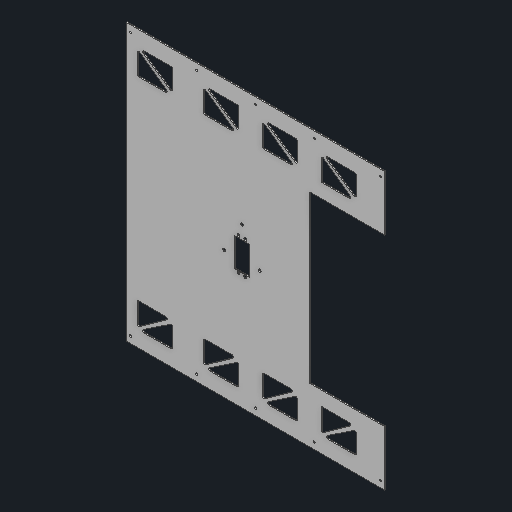
# Autodesk Inventor part: ВЕРХ 25-26
Saved by Autodesk Inventor 2026.2 (Build 302298000, 298)
## iProperties
Created: 2025-09-28
Part Number: ВЕРХ 25-26
Material: Типовые
Document SubType Name: Modeling
Designer: GameHD
Density: 1 g/cm^3
Appearance: По умолчанию
Author: GameHD
Autodesk Inventor part; units mm, degrees
(part 1 of 2)
ref_plane "YZ Plane" through (0, 0, 0) normal (1, 0, 0) x (0, 1, 0)
ref_plane "XZ Plane" through (0, 0, 0) normal (0, 1, 0) x (-1, 0, 0)
ref_plane "XY Plane" through (0, 0, 0) normal (0, 0, 1) x (1, 0, 0)
sketch "Эскиз1" plane through (0, 0, 0) normal (0, 0, 1) x (1, 0, 0)
  line L0 (0, 0) -> (380, 0)
  line L1 (380, 0) -> (380, 406)
  line L2 (380, 406) -> (0, 406)
  line L3 (0, 406) -> (0, 0)
  circle A0 centre (189.9999, 9.5) radius 1.625
  circle A1 centre (276.4236, 9.5) radius 1.625
  circle A2 centre (103.5763, 9.5) radius 1.625
  circle A3 centre (373.8998, 9.5) radius 1.625
  circle A4 centre (6.1, 9.5) radius 1.625
  line L4 (0, -31.725) -> (0, 41.275)
  line L5 (0, 203) -> (417.5125, 203)
  circle A5 centre (189.9999, 396.5) radius 1.625
  circle A6 centre (276.4236, 396.5) radius 1.625
  circle A7 centre (373.8998, 396.5) radius 1.625
  circle A8 centre (103.5763, 396.5) radius 1.625
  circle A9 centre (6.1, 396.5) radius 1.625
  circle A10 centre (189.9999, -129.0468) radius 1.625
  circle A11 centre (276.4236, -129.0468) radius 1.625
  circle A12 centre (373.8998, -129.0468) radius 1.625
  circle A13 centre (103.5763, -129.0468) radius 1.625
  circle A14 centre (6.1, -129.0468) radius 1.625
  circle A15 centre (189.9999, 535.0468) radius 1.625
  circle A16 centre (103.5763, 535.0468) radius 1.625
  circle A17 centre (373.8998, 535.0468) radius 1.625
  circle A18 centre (6.1, 535.0468) radius 1.625
  circle A19 centre (276.4236, 535.0468) radius 1.625
  line L6 (380, 203) -> (280, 203)
  line L7 (280, 203) -> (280, 81)
  line L8 (280, 81) -> (380, 81)
  line L9 (380, 81) -> (380, 203)
  line L10 (280, 203) -> (280, 325)
  line L11 (280, 325) -> (380, 325)
  circle A20 centre (6.1, 198.6) radius 1.625 projected
  arc A21 (257.5001, 181.25) -> (253.5001, 185.25) centre (253.5001, 181.25) ccw projected
  line L12 (253.5001, 185.25) -> (186.5001, 185.25) projected
  arc A22 (186.5001, 185.25) -> (182.5001, 181.25) centre (186.5001, 181.25) ccw projected
  line L13 (182.5001, 181.25) -> (182.5001, 139.25) projected
  arc A23 (182.5001, 139.25) -> (186.5001, 135.25) centre (186.5001, 139.25) ccw projected
  line L14 (186.5001, 135.25) -> (253.5001, 135.25) projected
  arc A24 (253.5001, 135.25) -> (257.5001, 139.25) centre (253.5001, 139.25) ccw projected
  line L15 (257.5001, 139.25) -> (257.5001, 181.25) projected
  line L16 (253.5001, -135.25) -> (186.5001, -135.25) projected
  arc A25 (186.5001, -135.25) -> (182.5001, -139.25) centre (186.5001, -139.25) ccw projected
  line L17 (182.5001, -139.25) -> (182.5001, -181.25) projected
  arc A26 (182.5001, -181.25) -> (186.5001, -185.25) centre (186.5001, -181.25) ccw projected
  line L18 (186.5001, -185.25) -> (253.5001, -185.25) projected
  arc A27 (253.5001, -185.25) -> (257.5001, -181.25) centre (253.5001, -181.25) ccw projected
  line L19 (257.5001, -181.25) -> (257.5001, -139.25) projected
  arc A28 (257.5001, -139.25) -> (253.5001, -135.25) centre (253.5001, -139.25) ccw projected
  arc A29 (148.6202, 128.9218) -> (145.3798, 128.9218) centre (147, 129.0468) ccw projected
  arc A30 (145.3798, 128.9218) -> (148.6202, 128.9218) centre (147, 128.7968) ccw projected
  arc A31 (371.3798, 111.6718) -> (374.6202, 111.6718) centre (373, 111.5468) ccw projected
  arc A32 (374.6202, 111.6718) -> (371.3798, 111.6718) centre (373, 111.7968) ccw projected
  arc A33 (231.3798, -128.9218) -> (234.6202, -128.9218) centre (233, -129.0468) ccw projected
  arc A34 (234.6202, -128.9218) -> (231.3798, -128.9218) centre (233, -128.7968) ccw projected
  arc A35 (5.38, -128.9218) -> (8.6204, -128.9218) centre (7.0002, -129.0468) ccw projected
  arc A36 (8.6204, -128.9218) -> (5.38, -128.9218) centre (7.0002, -128.7968) ccw projected
  arc A37 (148.6202, -111.6718) -> (145.3798, -111.6718) centre (147, -111.5468) ccw projected
  arc A38 (145.3798, -111.6718) -> (148.6202, -111.6718) centre (147, -111.7968) ccw projected
  arc A39 (374.6202, -111.6718) -> (371.3798, -111.6718) centre (373, -111.5468) ccw projected
  arc A40 (371.3798, -111.6718) -> (374.6202, -111.6718) centre (373, -111.7968) ccw projected
  arc A41 (231.3798, 111.6718) -> (234.6202, 111.6718) centre (233, 111.5468) ccw projected
  arc A42 (234.6202, 111.6718) -> (231.3798, 111.6718) centre (233, 111.7968) ccw projected
  arc A43 (5.38, 111.6718) -> (8.6204, 111.6718) centre (7.0002, 111.5468) ccw projected
  arc A44 (8.6204, 111.6718) -> (5.38, 111.6718) centre (7.0002, 111.7968) ccw projected
  arc A45 (145.3798, 111.6718) -> (148.6202, 111.6718) centre (147, 111.5468) ccw projected
  arc A46 (148.6202, 111.6718) -> (145.3798, 111.6718) centre (147, 111.7968) ccw projected
  arc A47 (374.6202, 128.9218) -> (371.3798, 128.9218) centre (373, 129.0468) ccw projected
  arc A48 (371.3798, 128.9218) -> (374.6202, 128.9218) centre (373, 128.7968) ccw projected
  arc A49 (234.6202, -111.6718) -> (231.3798, -111.6718) centre (233, -111.5468) ccw projected
  arc A50 (231.3798, -111.6718) -> (234.6202, -111.6718) centre (233, -111.7968) ccw projected
  arc A51 (8.6204, -111.6718) -> (5.38, -111.6718) centre (7.0002, -111.5468) ccw projected
  arc A52 (5.38, -111.6718) -> (8.6204, -111.6718) centre (7.0002, -111.7968) ccw projected
  arc A53 (145.3798, -128.9218) -> (148.6202, -128.9218) centre (147, -129.0468) ccw projected
  arc A54 (148.6202, -128.9218) -> (145.3798, -128.9218) centre (147, -128.7968) ccw projected
  arc A55 (371.3798, -128.9218) -> (374.6202, -128.9218) centre (373, -129.0468) ccw projected
  arc A56 (374.6202, -128.9218) -> (371.3798, -128.9218) centre (373, -128.7968) ccw projected
  arc A57 (234.6202, 128.9218) -> (231.3798, 128.9218) centre (233, 129.0468) ccw projected
  arc A58 (231.3798, 128.9218) -> (234.6202, 128.9218) centre (233, 128.7968) ccw projected
  arc A59 (8.6204, 128.9218) -> (5.38, 128.9218) centre (7.0002, 129.0468) ccw projected
  arc A60 (5.38, 128.9218) -> (8.6204, 128.9218) centre (7.0002, 128.7968) ccw projected
  circle A61 centre (373.9, 198.6) radius 1.625 projected
  circle A62 centre (374, -198.6) radius 1.625 projected
  circle A63 centre (6.1, 198.6) radius 1.625 projected
  circle A64 centre (6.1, -198.6) radius 1.625 projected
  circle A65 centre (190.0848, 193.5) radius 1.625 projected
  circle A66 centre (190.0848, -193.5) radius 1.625 projected
  circle A67 centre (233, 193.5) radius 1.625 projected
  circle A68 centre (233, -193.5) radius 1.625 projected
  circle A69 centre (134.0059, -1.825) radius 1.85 projected
  arc A70 (197.7028, 0) -> (198.309, 0) centre (198.0059, -1.825) ccw projected
  line L20 (198.309, 0) -> (197.7028, 0) projected
  circle A71 centre (134.0059, -60.625) radius 2 projected
  circle A72 centre (317.9941, 32.25) radius 2.1 projected
  circle A73 centre (62.0059, -32.25) radius 2.1 projected
  circle A74 centre (123.0059, -32.25) radius 2.1 projected
  circle A75 centre (317.9941, -32.25) radius 2.1 projected
  circle A76 centre (256.9941, 32.25) radius 2.1 projected
  circle A77 centre (62.0059, 32.25) radius 2.1 projected
  circle A78 centre (123.0059, 32.25) radius 2.1 projected
  circle A79 centre (256.9941, -32.25) radius 2.1 projected
  line L21 (49, -20) -> (13, -20) projected
  arc A80 (13, -20) -> (10, -23) centre (13, -23) ccw projected
  line L22 (10, -23) -> (10, -89) projected
  arc A81 (10, -89) -> (13, -92) centre (13, -89) ccw projected
  line L23 (13, -92) -> (49, -92) projected
  arc A82 (49, -92) -> (52, -89) centre (49, -89) ccw projected
  line L24 (52, -89) -> (52, -23) projected
  arc A83 (52, -23) -> (49, -20) centre (49, -23) ccw projected
  circle A84 centre (170.0002, 134.1128) radius 2.1 projected
  circle A85 centre (61.343, 102) radius 2.1 projected
  circle A86 centre (170.0002, -134.1128) radius 2.1 projected
  circle A87 centre (61.343, -11.0092) radius 2.1 projected
  circle A88 centre (65, -49.75) radius 2.1 projected
  circle A89 centre (65, -82) radius 2.1 projected
  arc A90 (32.152, -145) -> (34.152, -143) centre (32.152, -143) ccw projected
  line L25 (32.152, -145) -> (8, -145) projected
  arc A91 (8, -145) -> (5, -148) centre (8, -148) ccw projected
  line L26 (5, -148) -> (5, -192) projected
  arc A92 (5, -192) -> (8, -195) centre (8, -192) ccw projected
  line L27 (8, -195) -> (165, -195) projected
  arc A93 (165, -195) -> (168, -192) centre (165, -192) ccw projected
  line L28 (168, -192) -> (168, -148) projected
  arc A94 (168, -148) -> (165, -145) centre (165, -148) ccw projected
  line L29 (165, -145) -> (116.152, -145) projected
  arc A95 (114.152, -143) -> (116.152, -145) centre (116.152, -143) ccw projected
  line L30 (114.152, -143) -> (114.152, -131) projected
  arc A96 (114.152, -131) -> (112.152, -129) centre (112.152, -131) ccw projected
  line L31 (112.152, -129) -> (36.152, -129) projected
  arc A97 (36.152, -129) -> (34.152, -131) centre (36.152, -131) ccw projected
  line L32 (34.152, -131) -> (34.152, -143) projected
  arc A98 (345.848, -143) -> (347.848, -145) centre (347.848, -143) ccw projected
  line L33 (345.848, -143) -> (345.848, -131) projected
  arc A99 (345.848, -131) -> (343.848, -129) centre (343.848, -131) ccw projected
  line L34 (343.848, -129) -> (267.848, -129) projected
  arc A100 (267.848, -129) -> (265.848, -131) centre (267.848, -131) ccw projected
  line L35 (265.848, -131) -> (265.848, -193) projected
  arc A101 (265.848, -193) -> (267.848, -195) centre (267.848, -193) ccw projected
  line L36 (267.848, -195) -> (372, -195) projected
  arc A102 (372, -195) -> (375, -192) centre (372, -192) ccw projected
  line L37 (375, -192) -> (375, -148) projected
  arc A103 (375, -148) -> (372, -145) centre (372, -148) ccw projected
  line L38 (372, -145) -> (347.848, -145) projected
  arc A104 (347.848, 145) -> (345.848, 143) centre (347.848, 143) ccw projected
  line L39 (347.848, 145) -> (372, 145) projected
  arc A105 (372, 145) -> (375, 148) centre (372, 148) ccw projected
  line L40 (375, 148) -> (375, 192) projected
  arc A106 (375, 192) -> (372, 195) centre (372, 192) ccw projected
  line L41 (372, 195) -> (267.848, 195) projected
  arc A107 (267.848, 195) -> (265.848, 193) centre (267.848, 193) ccw projected
  line L42 (265.848, 193) -> (265.848, 131) projected
  arc A108 (265.848, 131) -> (267.848, 129) centre (267.848, 131) ccw projected
  line L43 (267.848, 129) -> (343.848, 129) projected
  arc A109 (343.848, 129) -> (345.848, 131) centre (343.848, 131) ccw projected
  line L44 (345.848, 131) -> (345.848, 143) projected
  arc A110 (34.152, 143) -> (32.152, 145) centre (32.152, 143) ccw projected
  line L45 (34.152, 143) -> (34.152, 131) projected
  arc A111 (34.152, 131) -> (36.152, 129) centre (36.152, 131) ccw projected
  line L46 (36.152, 129) -> (112.152, 129) projected
  arc A112 (112.152, 129) -> (114.152, 131) centre (112.152, 131) ccw projected
  line L47 (114.152, 131) -> (114.152, 143) projected
  arc A113 (116.152, 145) -> (114.152, 143) centre (116.152, 143) ccw projected
  line L48 (116.152, 145) -> (165, 145) projected
  arc A114 (165, 145) -> (168, 148) centre (165, 148) ccw projected
  line L49 (168, 148) -> (168, 192) projected
  arc A115 (168, 192) -> (165, 195) centre (165, 192) ccw projected
  line L50 (165, 195) -> (8, 195) projected
  arc A116 (8, 195) -> (5, 192) centre (8, 192) ccw projected
  line L51 (5, 192) -> (5, 148) projected
  arc A117 (5, 148) -> (8, 145) centre (8, 148) ccw projected
  line L52 (8, 145) -> (32.152, 145) projected
  line L53 (176.1539, 5.9063) -> (141.4028, 21.6949) projected
  arc A118 (141.4028, 21.6949) -> (137.8279, 17.0788) centre (140.1619, 18.9636) ccw projected
  line L54 (137.8279, 17.0788) -> (150.5778, 1.2902) projected
  arc A119 (150.5778, 1.2902) -> (152.9118, 0.175) centre (152.9118, 3.175) ccw projected
  line L55 (152.9118, 0.175) -> (174.913, 0.175) projected
  arc A120 (174.913, 0.175) -> (176.1539, 5.9063) centre (174.913, 3.175) ccw projected
  line L56 (164.9717, -29.4592) -> (165.9394, -28.5702) projected
  arc A121 (165.9394, -28.5702) -> (166.2437, -24.4762) centre (163.9097, -26.361) ccw projected
  line L57 (166.2437, -24.4762) -> (150.4677, -4.9402) projected
  arc A122 (150.4677, -4.9402) -> (148.1337, -3.825) centre (148.1337, -6.825) ccw projected
  line L58 (148.1337, -3.825) -> (145.4623, -3.825) projected
  arc A123 (145.4623, -3.825) -> (142.7128, -5.625) centre (145.4623, -6.825) ccw projected
  arc A124 (137.8059, -10.5319) -> (142.7128, -5.625) centre (134.0059, -1.825) ccw projected
  arc A125 (137.8059, -10.5319) -> (136.0059, -13.2814) centre (139.0059, -13.2814) ccw projected
  line L59 (136.0059, -13.2814) -> (136.0059, -27.25) projected
  arc A126 (136.0059, -27.25) -> (139.0059, -30.25) centre (139.0059, -27.25) ccw projected
  line L60 (139.0059, -30.25) -> (162.942, -30.25) projected
  arc A127 (162.942, -30.25) -> (164.9717, -29.4592) centre (162.942, -27.25) ccw projected
  line L61 (190.9762, -10.9995) -> (175.6931, -25.0408) projected
  arc A128 (175.6931, -25.0408) -> (177.7227, -30.25) centre (177.7227, -27.25) ccw projected
  line L62 (177.7227, -30.25) -> (193.0059, -30.25) projected
  arc A129 (193.0059, -30.25) -> (196.0059, -27.25) centre (193.0059, -27.25) ccw projected
  line L63 (196.0059, -27.25) -> (196.0059, -13.2086) projected
  arc A130 (196.0059, -13.2086) -> (190.9762, -10.9995) centre (193.0059, -13.2086) ccw projected
  line L64 (75.0034, -76.8076) -> (112.8628, -65.0804) projected
  arc A131 (112.8628, -65.0804) -> (112.4422, -59.2513) centre (111.9752, -62.2148) ccw projected
  line L65 (112.4422, -59.2513) -> (74.5828, -53.2849) projected
  arc A132 (74.5828, -53.2849) -> (71.1158, -56.2483) centre (74.1158, -56.2483) ccw projected
  line L66 (71.1158, -56.2483) -> (71.1158, -73.942) projected
  arc A133 (71.1158, -73.942) -> (75.0034, -76.8076) centre (74.1158, -73.942) ccw projected
  line L67 (273.1271, 34.25) -> (305.3345, 34.25) projected
  arc A134 (305.3345, 34.25) -> (307.3845, 39.4403) centre (305.3345, 37.25) ccw projected
  line L68 (307.3845, 39.4403) -> (293.7654, 52.1866) projected
  arc A135 (293.7654, 52.1866) -> (290.0188, 52.4704) centre (291.7154, 49.9963) ccw projected
  line L69 (290.0188, 52.4704) -> (271.4305, 39.7242) projected
  arc A136 (271.4305, 39.7242) -> (273.1271, 34.25) centre (273.1271, 37.25) ccw projected
  line L70 (237.7677, -24.5838) -> (207.2709, -8.8541) projected
  arc A137 (207.2709, -8.8541) -> (204.0022, -9.1935) centre (205.8957, -11.5203) ccw projected
  arc A138 (201.8059, -10.5319) -> (204.0022, -9.1935) centre (198.0059, -1.825) ccw projected
  arc A139 (201.8059, -10.5319) -> (200.0059, -13.2814) centre (203.0059, -13.2814) ccw projected
  line L71 (200.0059, -13.2814) -> (200.0059, -27.25) projected
  arc A140 (200.0059, -27.25) -> (203.0059, -30.25) centre (203.0059, -27.25) ccw projected
  line L72 (203.0059, -30.25) -> (236.3925, -30.25) projected
  arc A141 (236.3925, -30.25) -> (237.7677, -24.5838) centre (236.3925, -27.25) ccw projected
  line L73 (171.7502, 96.3659) -> (188.242, 84.4391) projected
  arc A142 (188.242, 84.4391) -> (191.758, 84.4391) centre (190, 86.8701) ccw projected
  line L74 (191.758, 84.4391) -> (215.7595, 101.7968) projected
  line L75 (215.7595, 101.7968) -> (173.5082, 101.7968) projected
  arc A143 (173.5082, 101.7968) -> (171.7502, 96.3659) centre (173.5082, 98.7968) ccw projected
  line L76 (265.3115, 40.3784) -> (285.9348, 54.5201) projected
  arc A144 (285.9348, 54.5201) -> (286.2882, 59.1846) centre (284.2382, 56.9942) ccw projected
  line L77 (286.2882, 59.1846) -> (245.2049, 97.6348) projected
  arc A145 (245.2049, 97.6348) -> (240.2828, 94.5781) centre (243.1549, 95.4444) ccw projected
  line L78 (240.2828, 94.5781) -> (255.6005, 43.7959) projected
  arc A146 (255.6005, 43.7959) -> (258.1178, 41.6833) centre (258.4726, 44.6622) ccw projected
  arc A147 (262.0259, 40.308) -> (258.1178, 41.6833) centre (256.9941, 32.25) ccw projected
  arc A148 (262.0259, 40.308) -> (265.3115, 40.3784) centre (263.6149, 42.8526) ccw projected
  arc A149 (72.6155, 39.4403) -> (74.6655, 34.25) centre (74.6655, 37.25) ccw projected
  line L79 (74.6655, 34.25) -> (111.9119, 34.25) projected
  arc A150 (111.9119, 34.25) -> (114.1595, 39.237) centre (111.9119, 37.25) ccw projected
  line L80 (114.1595, 39.237) -> (97.2953, 58.3129) projected
  arc A151 (97.2953, 58.3129) -> (92.9977, 58.5163) centre (95.0477, 56.3259) ccw projected
  line L81 (92.9977, 58.5163) -> (72.6155, 39.4403) projected
  line L82 (252.1574, 96.6064) -> (290.6344, 60.5955) projected
  arc A152 (290.6344, 60.5955) -> (294.3809, 60.3117) centre (292.6843, 62.7859) ccw projected
  line L83 (294.3809, 60.3117) -> (316.6907, 75.6098) projected
  arc A153 (316.6907, 75.6098) -> (317.9941, 78.084) centre (314.9941, 78.084) ccw projected
  line L84 (317.9941, 78.084) -> (317.9941, 98.7968) projected
  arc A154 (317.9941, 98.7968) -> (314.9941, 101.7968) centre (314.9941, 98.7968) ccw projected
  line L85 (314.9941, 101.7968) -> (254.2074, 101.7968) projected
  arc A155 (254.2074, 101.7968) -> (252.1574, 96.6064) centre (254.2074, 98.7968) ccw projected
  line L86 (196.7743, 78.2686) -> (212.8517, 66.6416) projected
  arc A156 (212.8517, 66.6416) -> (217.4768, 68.1895) centre (214.6097, 69.0726) ccw projected
  line L87 (217.4768, 68.1895) -> (226.6315, 97.9138) projected
  arc A157 (226.6315, 97.9138) -> (223.7644, 101.7968) centre (223.7644, 98.7968) ccw projected
  line L88 (223.7644, 101.7968) -> (223.5564, 101.7968) projected
  arc A158 (223.5564, 101.7968) -> (221.7984, 101.2277) centre (223.5564, 98.7968) ccw projected
  line L89 (221.7984, 101.2277) -> (196.7743, 83.1305) projected
  arc A159 (196.7743, 83.1305) -> (196.7743, 78.2686) centre (198.5323, 80.6996) ccw projected
  line L90 (209.1045, -5.2991) -> (247.729, -25.2209) projected
  arc A160 (247.729, -25.2209) -> (250.9978, -24.8815) centre (249.1042, -22.5547) ccw projected
  arc A161 (253.1941, -23.5431) -> (250.9978, -24.8815) centre (256.9941, -32.25) ccw projected
  arc A162 (253.1941, -23.5431) -> (254.9941, -20.7936) centre (251.9941, -20.7936) ccw projected
  line L91 (254.9941, -20.7936) -> (254.9941, 20.7936) projected
  arc A163 (254.9941, 20.7936) -> (253.1941, 23.5431) centre (251.9941, 20.7936) ccw projected
  arc A164 (251.3555, 24.6044) -> (253.1941, 23.5431) centre (256.9941, 32.25) ccw projected
  arc A165 (251.3555, 24.6044) -> (248.0743, 24.7877) centre (249.5749, 22.1899) ccw projected
  line L92 (248.0743, 24.7877) -> (208.9265, 2.1737) projected
  arc A166 (208.9265, 2.1737) -> (207.446, -0.7603) centre (210.4271, -0.424) ccw projected
  arc A167 (207.486, -2.439) -> (207.446, -0.7603) centre (198.0059, -1.825) ccw projected
  arc A168 (207.486, -2.439) -> (209.1045, -5.2991) centre (210.4797, -2.6329) ccw projected
  line L93 (290.6344, -60.5955) -> (250.0205, -98.6064) projected
  arc A169 (250.0205, -98.6064) -> (252.0705, -103.7968) centre (252.0705, -100.7968) ccw projected
  line L94 (252.0705, -103.7968) -> (314.9941, -103.7968) projected
  arc A170 (314.9941, -103.7968) -> (317.9941, -100.7968) centre (314.9941, -100.7968) ccw projected
  line L95 (317.9941, -100.7968) -> (317.9941, -78.084) projected
  arc A171 (317.9941, -78.084) -> (316.6907, -75.6098) centre (314.9941, -78.084) ccw projected
  line L96 (316.6907, -75.6098) -> (294.3809, -60.3117) projected
  arc A172 (294.3809, -60.3117) -> (290.6344, -60.5955) centre (292.6843, -62.7859) ccw projected
  line L97 (258.9941, 19.6864) -> (258.9941, -19.6864) projected
  arc A173 (258.9941, -19.6864) -> (264.1737, -21.7477) centre (261.9941, -19.6864) ccw projected
  line L98 (264.1737, -21.7477) -> (282.7918, -2.0614) projected
  arc A174 (282.7918, -2.0614) -> (282.7918, 2.0614) centre (280.6122, 0) ccw projected
  line L99 (282.7918, 2.0614) -> (264.1737, 21.7477) projected
  arc A175 (264.1737, 21.7477) -> (258.9941, 19.6864) centre (261.9941, 19.6864) ccw projected
  line L100 (73.6488, -49.0883) -> (89.4125, -51.5726) projected
  arc A176 (89.4125, -51.5726) -> (90.9794, -45.8181) centre (89.8795, -48.6092) ccw projected
  line L101 (90.9794, -45.8181) -> (75.2157, -39.6057) projected
  arc A177 (75.2157, -39.6057) -> (71.1158, -42.3967) centre (74.1158, -42.3967) ccw projected
  line L102 (71.1158, -42.3967) -> (71.1158, -46.1249) projected
  arc A178 (71.1158, -46.1249) -> (73.6488, -49.0883) centre (74.1158, -46.1249) ccw projected
  line L103 (136.0059, -37.25) -> (136.0059, -49.2414) projected
  arc A179 (136.0059, -49.2414) -> (141.0355, -51.4505) centre (139.0059, -49.2414) ccw projected
  line L104 (141.0355, -51.4505) -> (154.0874, -39.4592) projected
  arc A180 (154.0874, -39.4592) -> (152.0577, -34.25) centre (152.0577, -37.25) ccw projected
  line L105 (152.0577, -34.25) -> (139.0059, -34.25) projected
  arc A181 (139.0059, -34.25) -> (136.0059, -37.25) centre (139.0059, -37.25) ccw projected
  line L106 (187.6976, 26.0214) -> (194.3962, 11.0995) projected
  arc A182 (194.3962, 11.0995) -> (200.0002, 11.4451) centre (197.1331, 12.3281) ccw projected
  line L107 (200.0002, 11.4451) -> (204.5959, 26.367) projected
  arc A183 (204.5959, 26.367) -> (201.7288, 30.25) centre (201.7288, 27.25) ccw projected
  line L108 (201.7288, 30.25) -> (190.4345, 30.25) projected
  arc A184 (190.4345, 30.25) -> (187.6976, 26.0214) centre (190.4345, 27.25) ccw projected
  line L109 (96.148, -15.0552) -> (84.8346, -0.4618) projected
  arc A185 (84.8346, -0.4618) -> (80.7407, 0.156) centre (82.4637, -2.2999) ccw projected
  line L110 (80.7407, 0.156) -> (72.3928, -5.7004) projected
  arc A186 (72.3928, -5.7004) -> (71.1158, -8.1563) centre (74.1158, -8.1563) ccw projected
  line L111 (71.1158, -8.1563) -> (71.1158, -10.1207) projected
  arc A187 (71.1158, -10.1207) -> (73.1387, -12.9571) centre (74.1158, -10.1207) ccw projected
  line L112 (73.1387, -12.9571) -> (92.8, -19.7297) projected
  arc A188 (92.8, -19.7297) -> (96.148, -15.0552) centre (93.777, -16.8933) ccw projected
  line L113 (158.6531, -8.7098) -> (168.9546, -21.4664) projected
  arc A189 (168.9546, -21.4664) -> (173.3182, -21.7908) centre (171.2886, -19.5816) ccw projected
  line L114 (173.3182, -21.7908) -> (187.203, -9.0342) projected
  arc A190 (187.203, -9.0342) -> (185.1733, -3.825) centre (185.1733, -6.825) ccw projected
  line L115 (185.1733, -3.825) -> (160.9871, -3.825) projected
  arc A191 (160.9871, -3.825) -> (158.6531, -8.7098) centre (160.9871, -6.825) ccw projected
  line L116 (88.7233, 10.6423) -> (108.8956, 24.7941) projected
  arc A192 (108.8956, 24.7941) -> (107.1727, 30.25) centre (107.1727, 27.25) ccw projected
  line L117 (107.1727, 30.25) -> (74.1158, 30.25) projected
  arc A193 (74.1158, 30.25) -> (71.1158, 27.25) centre (74.1158, 27.25) ccw projected
  line L118 (71.1158, 27.25) -> (71.1158, 26.722) projected
  arc A194 (71.1158, 26.722) -> (71.9361, 24.6607) centre (74.1158, 26.722) ccw projected
  line L119 (71.9361, 24.6607) -> (84.8207, 11.0368) projected
  arc A195 (84.8207, 11.0368) -> (88.7233, 10.6423) centre (87.0003, 13.0982) ccw projected
  line L120 (138.452, 34.25) -> (174.984, 34.25) projected
  arc A196 (174.984, 34.25) -> (177.7209, 38.4786) centre (174.984, 37.25) ccw projected
  line L121 (177.7209, 38.4786) -> (168.7676, 58.4233) projected
  arc A197 (168.7676, 58.4233) -> (164.2727, 59.6256) centre (166.0307, 57.1947) ccw projected
  line L122 (164.2727, 59.6256) -> (136.694, 39.6809) projected
  arc A198 (136.694, 39.6809) -> (138.452, 34.25) centre (138.452, 37.25) ccw projected
  line L123 (183.2224, -39.1348) -> (190.6719, -48.3597) projected
  arc A199 (190.6719, -48.3597) -> (196.0059, -46.4749) centre (193.0059, -46.4749) ccw projected
  line L124 (196.0059, -46.4749) -> (196.0059, -37.25) projected
  arc A200 (196.0059, -37.25) -> (193.0059, -34.25) centre (193.0059, -37.25) ccw projected
  line L125 (193.0059, -34.25) -> (185.5564, -34.25) projected
  arc A201 (185.5564, -34.25) -> (183.2224, -39.1348) centre (185.5564, -37.25) ccw projected
  line L126 (104.4945, -94.2234) -> (129.3603, -103.259) projected
  arc A202 (129.3603, -103.259) -> (133.3849, -100.4394) centre (130.3849, -100.4394) ccw projected
  line L127 (133.3849, -100.4394) -> (133.3849, -94.0885) projected
  arc A203 (133.3849, -94.0885) -> (130.7069, -91.1058) centre (130.3849, -94.0885) ccw projected
  line L128 (130.7069, -91.1058) -> (105.8411, -88.4211) projected
  arc A204 (105.8411, -88.4211) -> (104.4945, -94.2234) centre (105.5191, -91.4038) ccw projected
  line L129 (266.425, 25.1886) -> (285.3145, 5.2154) projected
  arc A205 (285.3145, 5.2154) -> (289.6737, 5.2154) centre (287.4941, 7.2768) ccw projected
  line L130 (289.6737, 5.2154) -> (308.5632, 25.1886) projected
  arc A206 (308.5632, 25.1886) -> (306.3835, 30.25) centre (306.3835, 27.25) ccw projected
  line L131 (306.3835, 30.25) -> (268.6047, 30.25) projected
  arc A207 (268.6047, 30.25) -> (266.425, 25.1886) centre (268.6047, 27.25) ccw projected
  line L132 (76.1657, 48.2416) -> (90.4716, 61.6306) projected
  arc A208 (90.4716, 61.6306) -> (90.6693, 65.808) centre (88.4217, 63.821) ccw projected
  line L133 (90.6693, 65.808) -> (76.3634, 81.9901) projected
  arc A209 (76.3634, 81.9901) -> (71.1158, 80.0031) centre (74.1158, 80.0031) ccw projected
  line L134 (71.1158, 80.0031) -> (71.1158, 50.432) projected
  arc A210 (71.1158, 50.432) -> (76.1657, 48.2416) centre (74.1158, 50.432) ccw projected
  line L135 (133.824, 42.5418) -> (163.6065, 64.0802) projected
  arc A211 (163.6065, 64.0802) -> (164.5853, 67.7397) centre (161.8485, 66.5111) ccw projected
  line L136 (164.5853, 67.7397) -> (150.6579, 98.7648) projected
  arc A212 (150.6579, 98.7648) -> (145.0488, 98.4025) centre (147.921, 97.5362) ccw projected
  line L137 (145.0488, 98.4025) -> (129.1938, 45.8391) projected
  arc A213 (129.1938, 45.8391) -> (133.824, 42.5418) centre (132.066, 44.9727) ccw projected
  line L138 (71.8682, 93.1141) -> (93.4781, 68.6699) projected
  arc A214 (93.4781, 68.6699) -> (97.7757, 68.4666) centre (95.7258, 70.657) ccw projected
  line L139 (97.7757, 68.4666) -> (127.8426, 96.6064) projected
  arc A215 (127.8426, 96.6064) -> (125.7926, 101.7968) centre (125.7926, 98.7968) ccw projected
  line L140 (125.7926, 101.7968) -> (74.1158, 101.7968) projected
  arc A216 (74.1158, 101.7968) -> (71.1158, 98.7968) centre (74.1158, 98.7968) ccw projected
  line L141 (71.1158, 98.7968) -> (71.1158, 95.1011) projected
  arc A217 (71.1158, 95.1011) -> (71.8682, 93.1141) centre (74.1158, 95.1011) ccw projected
  line L142 (243.306, 39.6809) -> (221.8167, 55.2218) projected
  arc A218 (221.8167, 55.2218) -> (217.1916, 53.6739) centre (220.0587, 52.7909) ccw projected
  line L143 (217.1916, 53.6739) -> (212.4052, 38.133) projected
  arc A219 (212.4052, 38.133) -> (215.2723, 34.25) centre (215.2723, 37.25) ccw projected
  line L144 (215.2723, 34.25) -> (241.548, 34.25) projected
  arc A220 (241.548, 34.25) -> (243.306, 39.6809) centre (241.548, 37.25) ccw projected
  line L145 (207.6758, 36.367) -> (214.3683, 58.0966) projected
  arc A221 (214.3683, 58.0966) -> (213.2592, 61.4105) centre (211.5012, 58.9796) ccw projected
  line L146 (213.2592, 61.4105) -> (191.758, 76.96) projected
  arc A222 (191.758, 76.96) -> (188.242, 76.96) centre (190, 74.529) ccw projected
  line L147 (188.242, 76.96) -> (172.5476, 65.6099) projected
  arc A223 (172.5476, 65.6099) -> (171.5688, 61.9504) centre (174.3056, 63.179) ccw projected
  line L148 (171.5688, 61.9504) -> (183.2085, 36.0214) projected
  arc A224 (183.2085, 36.0214) -> (185.9454, 34.25) centre (185.9454, 37.25) ccw projected
  line L149 (185.9454, 34.25) -> (204.8087, 34.25) projected
  arc A225 (204.8087, 34.25) -> (207.6758, 36.367) centre (204.8087, 37.25) ccw projected
  line L150 (285.3145, -5.2154) -> (266.425, -25.1886) projected
  arc A226 (266.425, -25.1886) -> (268.6047, -30.25) centre (268.6047, -27.25) ccw projected
  line L151 (268.6047, -30.25) -> (306.3835, -30.25) projected
  arc A227 (306.3835, -30.25) -> (308.5632, -25.1886) centre (306.3835, -27.25) ccw projected
  line L152 (308.5632, -25.1886) -> (289.6737, -5.2154) projected
  arc A228 (289.6737, -5.2154) -> (285.3145, -5.2154) centre (287.4941, -7.2768) ccw projected
  line L153 (310.8145, 21.7477) -> (292.1964, 2.0614) projected
  arc A229 (292.1964, 2.0614) -> (292.1964, -2.0614) centre (294.376, 0) ccw projected
  line L154 (292.1964, -2.0614) -> (310.8145, -21.7477) projected
  arc A230 (310.8145, -21.7477) -> (315.9941, -19.6864) centre (312.9941, -19.6864) ccw projected
  line L155 (315.9941, -19.6864) -> (315.9941, 19.6864) projected
  arc A231 (315.9941, 19.6864) -> (310.8145, 21.7477) centre (312.9941, 19.6864) ccw projected
  line L156 (190.7609, 9.4306) -> (182.21, 28.4786) projected
  arc A232 (182.21, 28.4786) -> (179.4731, 30.25) centre (179.4731, 27.25) ccw projected
  line L157 (179.4731, 30.25) -> (146.0987, 30.25) projected
  arc A233 (146.0987, 30.25) -> (144.8578, 24.5187) centre (146.0987, 27.25) ccw projected
  line L158 (144.8578, 24.5187) -> (186.783, 5.4706) projected
  arc A234 (186.783, 5.4706) -> (190.7609, 9.4306) centre (188.024, 8.202) ccw projected
  line L159 (121.268, -47.4583) -> (111.9292, -35.4119) projected
  arc A235 (111.9292, -35.4119) -> (109.5582, -34.25) centre (109.5582, -37.25) ccw projected
  line L160 (109.5582, -34.25) -> (88.33, -34.25) projected
  arc A236 (88.33, -34.25) -> (87.2301, -40.0411) centre (88.33, -37.25) ccw projected
  line L161 (87.2301, -40.0411) -> (117.797, -52.0874) projected
  arc A237 (117.797, -52.0874) -> (121.268, -47.4583) centre (118.897, -49.2964) ccw projected
  line L162 (114.7758, 24.0332) -> (92.2222, 8.2108) projected
  arc A238 (92.2222, 8.2108) -> (91.7655, 3.6935) centre (93.9452, 5.7549) ccw projected
  line L163 (91.7655, 3.6935) -> (115.8263, -21.7477) projected
  arc A239 (115.8263, -21.7477) -> (121.0059, -19.6864) centre (118.0059, -19.6864) ccw projected
  line L164 (121.0059, -19.6864) -> (121.0059, 20.7936) projected
  arc A240 (121.0059, 20.7936) -> (119.2059, 23.5431) centre (118.0059, 20.7936) ccw projected
  arc A241 (118.0605, 24.1387) -> (119.2059, 23.5431) centre (123.0059, 32.25) ccw projected
  arc A242 (118.0605, 24.1387) -> (114.7758, 24.0332) centre (116.4988, 21.5773) ccw projected
  line L165 (285.9348, -54.5201) -> (283.4292, -52.8019) projected
  arc A243 (283.4292, -52.8019) -> (280.4301, -52.5736) centre (281.7326, -55.2761) ccw projected
  line L166 (280.4301, -52.5736) -> (242.0824, -71.0547) projected
  arc A244 (242.0824, -71.0547) -> (240.3849, -73.7572) centre (243.3849, -73.7572) ccw projected
  line L167 (240.3849, -73.7572) -> (240.3849, -95.2293) projected
  arc A245 (240.3849, -95.2293) -> (245.4348, -97.4196) centre (243.3849, -95.2293) ccw projected
  line L168 (245.4348, -97.4196) -> (286.2882, -59.1846) projected
  arc A246 (286.2882, -59.1846) -> (285.9348, -54.5201) centre (284.2382, -56.9942) ccw projected
  line L169 (139.3849, -79.25) -> (139.3849, -103.25) projected
  arc A247 (139.3849, -103.25) -> (142.3849, -106.25) centre (142.3849, -103.25) ccw projected
  line L170 (142.3849, -106.25) -> (231.3849, -106.25) projected
  arc A248 (231.3849, -106.25) -> (234.3849, -103.25) centre (231.3849, -103.25) ccw projected
  line L171 (234.3849, -103.25) -> (234.3849, -79.25) projected
  arc A249 (234.3849, -79.25) -> (231.3849, -76.25) centre (231.3849, -79.25) ccw projected
  line L172 (231.3849, -76.25) -> (142.3849, -76.25) projected
  arc A250 (142.3849, -76.25) -> (139.3849, -79.25) centre (142.3849, -79.25) ccw projected
  line L173 (134.7951, 97.6348) -> (100.3018, 65.3522) projected
  arc A251 (100.3018, 65.3522) -> (100.1042, 61.1749) centre (102.3518, 63.1619) ccw projected
  line L174 (100.1042, 61.1749) -> (116.9163, 42.1579) projected
  arc A252 (116.9163, 42.1579) -> (120.086, 41.2901) centre (119.1639, 44.1449) ccw projected
  arc A253 (121.8822, 41.6833) -> (120.086, 41.2901) centre (123.0059, 32.25) ccw projected
  arc A254 (121.8822, 41.6833) -> (124.3995, 43.7959) centre (121.5274, 44.6622) ccw projected
  line L175 (124.3995, 43.7959) -> (139.7172, 94.5781) projected
  arc A255 (139.7172, 94.5781) -> (134.7951, 97.6348) centre (136.8451, 95.4444) ccw projected
  arc A256 (133.3849, -73.7642) -> (133.1423, -71.8089) centre (125.3849, -73.7642) ccw projected
  arc A257 (133.1423, -71.8089) -> (131.1387, -69.682) centre (130.2332, -72.5421) ccw projected
  arc A258 (126.839, -66.8608) -> (131.1387, -69.682) centre (134.0059, -60.625) ccw projected
  arc A259 (126.839, -66.8608) -> (124.0903, -65.8696) centre (124.5758, -68.8301) ccw projected
  arc A260 (124.0903, -65.8696) -> (123.0178, -66.1224) centre (125.3849, -73.7642) ccw projected
  line L176 (123.0178, -66.1224) -> (88.6823, -76.758) projected
  arc A261 (88.6823, -76.758) -> (89.2479, -82.6063) centre (89.57, -79.6237) ccw projected
  line L177 (89.2479, -82.6063) -> (130.0629, -87.013) projected
  arc A262 (130.0629, -87.013) -> (133.3849, -84.0303) centre (130.3849, -84.0303) ccw projected
  line L178 (133.3849, -84.0303) -> (133.3849, -73.7642) projected
  line L179 (94.1155, -24.4136) -> (75.0928, -17.8609) projected
  arc A263 (75.0928, -17.8609) -> (71.1158, -20.6973) centre (74.1158, -20.6973) ccw projected
  line L180 (71.1158, -20.6973) -> (71.1158, -27.25) projected
  arc A264 (71.1158, -27.25) -> (74.1158, -30.25) centre (74.1158, -27.25) ccw projected
  line L181 (74.1158, -30.25) -> (93.1384, -30.25) projected
  arc A265 (93.1384, -30.25) -> (94.1155, -24.4136) centre (93.1384, -27.25) ccw projected
  line L182 (230.0831, 95.5311) -> (220.3001, 63.7669) projected
  arc A266 (220.3001, 63.7669) -> (221.4092, 60.4529) centre (223.1672, 62.8838) ccw projected
  line L183 (221.4092, 60.4529) -> (246.176, 42.5418) projected
  arc A267 (246.176, 42.5418) -> (250.8062, 45.8391) centre (247.934, 44.9727) ccw projected
  line L184 (250.8062, 45.8391) -> (235.8223, 95.5144) projected
  arc A268 (235.8223, 95.5144) -> (230.0831, 95.5311) centre (232.9502, 94.648) ccw projected
  arc A269 (189.299, -64.425) -> (189.9499, -65.66) centre (198.0059, -60.625) ccw projected
  arc A270 (189.299, -64.425) -> (186.5494, -62.625) centre (186.5494, -65.625) ccw projected
  line L185 (186.5494, -62.625) -> (150.91, -62.625) projected
  arc A271 (150.91, -62.625) -> (149.278, -68.1423) centre (150.91, -65.625) ccw projected
  line L186 (149.278, -68.1423) -> (151.7846, -69.7673) projected
  arc A272 (151.7846, -69.7673) -> (153.4165, -70.25) centre (153.4165, -67.25) ccw projected
  line L187 (153.4165, -70.25) -> (187.4059, -70.25) projected
  arc A273 (187.4059, -70.25) -> (189.9499, -65.66) centre (187.4059, -67.25) ccw projected
  arc A274 (206.0618, -65.66) -> (207.3536, -62.3193) centre (198.0059, -60.625) ccw projected
  arc A275 (206.0618, -65.66) -> (208.6058, -70.25) centre (208.6058, -67.25) ccw projected
  line L188 (208.6058, -70.25) -> (233.8536, -70.25) projected
  arc A276 (233.8536, -70.25) -> (235.156, -69.9525) centre (233.8536, -67.25) ccw projected
  line L189 (235.156, -69.9525) -> (273.5281, -51.4596) projected
  arc A277 (273.5281, -51.4596) -> (273.9223, -46.2829) centre (272.2257, -48.7571) ccw projected
  line L190 (273.9223, -46.2829) -> (273.3304, -45.8771) projected
  arc A278 (273.3304, -45.8771) -> (270.9434, -45.4318) centre (271.6338, -48.3513) ccw projected
  line L191 (270.9434, -45.4318) -> (209.6151, -59.9348) projected
  arc A279 (209.6151, -59.9348) -> (207.3536, -62.3193) centre (210.3055, -62.8543) ccw projected
  line L192 (189.2522, -52.9684) -> (175.037, -35.3652) projected
  arc A280 (175.037, -35.3652) -> (172.703, -34.25) centre (172.703, -37.25) ccw projected
  line L193 (172.703, -34.25) -> (165.6695, -34.25) projected
  line L194 (165.6695, -34.25) -> (144.8087, -53.4158) projected
  arc A281 (144.8087, -53.4158) -> (146.8384, -58.625) centre (146.8384, -55.625) ccw projected
  line L195 (146.8384, -58.625) -> (186.5494, -58.625) projected
  arc A282 (186.5494, -58.625) -> (189.299, -56.825) centre (186.5494, -55.625) ccw projected
  arc A283 (189.5792, -56.2384) -> (189.299, -56.825) centre (198.0059, -60.625) ccw projected
  arc A284 (189.5792, -56.2384) -> (189.2522, -52.9684) centre (186.9182, -54.8532) ccw projected
  line L196 (207.463, -53.8565) -> (236.3657, -39.9535) projected
  arc A285 (236.3657, -39.9535) -> (235.0652, -34.25) centre (235.0652, -37.25) ccw projected
  line L197 (235.0652, -34.25) -> (203.0059, -34.25) projected
  arc A286 (203.0059, -34.25) -> (200.0059, -37.25) centre (203.0059, -37.25) ccw projected
  line L198 (200.0059, -37.25) -> (200.0059, -49.1686) projected
  arc A287 (200.0059, -49.1686) -> (201.8059, -51.9181) centre (203.0059, -49.1686) ccw projected
  arc A288 (204.2049, -53.4263) -> (201.8059, -51.9181) centre (198.0059, -60.625) ccw projected
  arc A289 (204.2049, -53.4263) -> (207.463, -53.8565) centre (206.1625, -51.153) ccw projected
  line L199 (238.3424, 30.25) -> (212.1924, 30.25) projected
  arc A290 (212.1924, 30.25) -> (209.3253, 28.133) centre (212.1924, 27.25) ccw projected
  line L200 (209.3253, 28.133) -> (203.666, 9.7581) projected
  arc A291 (203.666, 9.7581) -> (208.0337, 6.2774) centre (206.5331, 8.8751) ccw projected
  line L201 (208.0337, 6.2774) -> (239.843, 24.6523) projected
  arc A292 (239.843, 24.6523) -> (238.3424, 30.25) centre (238.3424, 27.25) ccw projected
  circle A293 centre (198.0059, -60.625) radius 2 projected
  line L202 (317.9941, 44.3847) -> (317.9941, 65.9588) projected
  arc A294 (317.9941, 65.9588) -> (313.2975, 68.433) centre (314.9941, 65.9588) ccw projected
  line L203 (313.2975, 68.433) -> (298.465, 58.2621) projected
  arc A295 (298.465, 58.2621) -> (298.1116, 53.5975) centre (300.1615, 55.7879) ccw projected
  line L204 (298.1116, 53.5975) -> (310.9962, 41.5387) projected
  arc A296 (310.9962, 41.5387) -> (314.2337, 40.9741) centre (313.0462, 43.729) ccw projected
  arc A297 (315.7141, 41.4723) -> (314.2337, 40.9741) centre (317.9941, 32.25) ccw projected
  arc A298 (315.7141, 41.4723) -> (317.9941, 44.3847) centre (314.9941, 44.3847) ccw projected
  line L205 (317.9941, -65.9588) -> (317.9941, -44.3847) projected
  arc A299 (317.9941, -44.3847) -> (315.7141, -41.4723) centre (314.9941, -44.3847) ccw projected
  arc A300 (314.2337, -40.9741) -> (315.7141, -41.4723) centre (317.9941, -32.25) ccw projected
  arc A301 (314.2337, -40.9741) -> (310.9962, -41.5387) centre (313.0462, -43.729) ccw projected
  line L206 (310.9962, -41.5387) -> (298.1116, -53.5975) projected
  arc A302 (298.1116, -53.5975) -> (298.465, -58.2621) centre (300.1615, -55.7879) ccw projected
  line L207 (298.465, -58.2621) -> (313.2975, -68.433) projected
  arc A303 (313.2975, -68.433) -> (317.9941, -65.9588) centre (314.9941, -65.9588) ccw projected
  line L208 (156.48, 95.5625) -> (167.3865, 71.2669) projected
  arc A304 (167.3865, 71.2669) -> (171.8814, 70.0646) centre (170.1234, 72.4955) ccw projected
  line L209 (171.8814, 70.0646) -> (183.2257, 78.2686) projected
  arc A305 (183.2257, 78.2686) -> (183.2257, 83.1305) centre (181.4677, 80.6996) ccw projected
  line L210 (183.2257, 83.1305) -> (160.9749, 99.2221) projected
  arc A306 (160.9749, 99.2221) -> (156.48, 95.5625) centre (159.2169, 96.7912) ccw projected
  circle A307 centre (5, -32.25) radius 1.5 projected
  circle A308 centre (5, -73.942) radius 1.5 projected
  line L211 (53.391, -10.921) -> (54.8002, -10.5715) projected
  arc A309 (54.8002, -10.5715) -> (56.8024, -8.9158) centre (54.078, -7.6597) ccw projected
  arc A310 (56.9059, -8.7045) -> (56.8024, -8.9158) centre (61.343, -11.0092) ccw projected
  arc A311 (56.9059, -8.7045) -> (56.987, -6.1077) centre (54.2436, -7.3217) ccw projected
  line L212 (56.987, -6.1077) -> (50.1126, 9.4273) projected
  arc A312 (50.1126, 9.4273) -> (45.1248, 10.204) centre (47.3692, 8.2133) ccw projected
  line L213 (45.1248, 10.204) -> (30.7357, -6.0185) projected
  arc A313 (30.7357, -6.0185) -> (32.98, -11.0092) centre (32.98, -8.0092) ccw projected
  line L214 (32.98, -11.0092) -> (52.6688, -11.0092) projected
  arc A314 (52.6688, -11.0092) -> (53.391, -10.921) centre (52.6688, -8.0092) ccw projected
  line L215 (41.1301, 58.9232) -> (35.4572, 67.1271) projected
  arc A315 (35.4572, 67.1271) -> (30.2462, 64.2069) centre (32.9896, 65.4209) ccw projected
  line L216 (30.2462, 64.2069) -> (34.9665, 53.5398) projected
  arc A316 (34.9665, 53.5398) -> (40.508, 53.6716) centre (37.7099, 54.7538) ccw projected
  line L217 (40.508, 53.6716) -> (41.4606, 56.1348) projected
  arc A317 (41.4606, 56.1348) -> (41.1301, 58.9232) centre (38.6625, 57.217) ccw projected
  line L218 (53.7933, 76.934) -> (47.1014, 59.631) projected
  arc A318 (47.1014, 59.631) -> (47.432, 56.8426) centre (49.8995, 58.5489) ccw projected
  line L219 (47.432, 56.8426) -> (54.3838, 46.7892) projected
  arc A319 (54.3838, 46.7892) -> (59.8512, 48.524) centre (56.8513, 48.4955) ccw projected
  line L220 (59.8512, 48.524) -> (59.5912, 75.8804) projected
  arc A320 (59.5912, 75.8804) -> (53.7933, 76.934) centre (56.5913, 75.8519) ccw projected
  arc A321 (57.2156, 33.683) -> (57.078, 31.4037) centre (62.0059, 32.25) ccw projected
  arc A322 (57.2156, 33.683) -> (56.809, 36.249) centre (54.3415, 34.5428) ccw projected
  line L221 (56.809, 36.249) -> (48.0061, 48.9794) projected
  arc A323 (48.0061, 48.9794) -> (42.7406, 48.3552) centre (45.5386, 47.2731) ccw projected
  line L222 (42.7406, 48.3552) -> (40.6333, 42.9064) projected
  arc A324 (40.6333, 42.9064) -> (40.6879, 40.6103) centre (43.4313, 41.8243) ccw projected
  line L223 (40.6879, 40.6103) -> (47.4724, 25.2787) projected
  arc A325 (47.4724, 25.2787) -> (52.4601, 24.5019) centre (50.2158, 26.4926) ccw projected
  line L224 (52.4601, 24.5019) -> (56.3657, 28.9052) projected
  arc A326 (56.3657, 28.9052) -> (57.078, 31.4037) centre (54.1213, 30.8959) ccw projected
  line L225 (54.5556, 20.8364) -> (52.4205, 18.4292) projected
  arc A327 (52.4205, 18.4292) -> (51.9214, 15.2245) centre (54.6648, 16.4385) ccw projected
  line L226 (51.9214, 15.2245) -> (53.9494, 10.6416) projected
  arc A328 (53.9494, 10.6416) -> (59.6925, 11.8096) centre (56.6928, 11.8556) ccw projected
  line L227 (59.6925, 11.8096) -> (59.7996, 18.7997) projected
  arc A329 (59.7996, 18.7997) -> (54.5556, 20.8364) centre (56.7999, 18.8457) ccw projected
  line L228 (10.1793, 85.3503) -> (10.1793, 1.601) projected
  arc A330 (10.1793, 1.601) -> (10.6534, -0.0176) centre (13.1793, 1.601) ccw projected
  arc A331 (10.6534, -0.0176) -> (18.3688, -1.5987) centre (15.2808, 2.9478) ccw projected
  arc A332 (18.3688, -1.5987) -> (19.7331, -0.0456) centre (16.9351, 1.0365) ccw projected
  line L229 (19.7331, -0.0456) -> (35.408, 40.4847) projected
  arc A333 (35.408, 40.4847) -> (35.3534, 42.7808) centre (32.61, 41.5668) ccw projected
  line L230 (35.3534, 42.7808) -> (15.9197, 86.6976) projected
  arc A334 (15.9197, 86.6976) -> (10.1793, 85.3503) centre (13.1763, 85.4837) ccw projected
  line L231 (45.8214, 67.4106) -> (57.2251, 96.8968) projected
  arc A335 (57.2251, 96.8968) -> (57.0205, 99.4869) centre (54.427, 97.979) ccw projected
  arc A336 (56.9474, 99.6171) -> (57.0205, 99.4869) centre (61.343, 102) ccw projected
  arc A337 (56.9474, 99.6171) -> (54.8423, 101.1397) centre (54.31, 98.1873) ccw projected
  line L232 (54.8423, 101.1397) -> (50.3342, 101.9524) projected
  arc A338 (50.3342, 101.9524) -> (49.8019, 102) centre (49.8019, 99) ccw projected
  line L233 (49.8019, 102) -> (21.928, 102) projected
  arc A339 (21.928, 102) -> (19.4605, 97.2937) centre (21.928, 99) ccw projected
  line L234 (19.4605, 97.2937) -> (40.5559, 66.7865) projected
  arc A340 (40.5559, 66.7865) -> (45.8214, 67.4106) centre (43.0234, 68.4928) ccw projected
  line L235 (29.9169, -0.9136) -> (45.1645, 16.2768) projected
  arc A341 (45.1645, 16.2768) -> (45.6635, 19.4814) centre (42.9201, 18.2675) ccw projected
  line L236 (45.6635, 19.4814) -> (41.0748, 29.8514) projected
  arc A342 (41.0748, 29.8514) -> (35.5333, 29.7195) centre (38.3314, 28.6374) ccw projected
  line L237 (35.5333, 29.7195) -> (24.8746, 2.1593) projected
  arc A343 (24.8746, 2.1593) -> (29.9169, -0.9136) centre (27.6726, 1.0771) ccw projected
  arc A344 (417.7779, 195.9889) -> (413.2002, 203) centre (413.2002, 198) ccw projected
  line L238 (417.7779, 195.9889) -> (380, 110) projected
  arc A345 (377, 107) -> (380, 110) centre (377, 110) ccw projected
  line L239 (377, 107) -> (326.5966, 107) projected
  line L240 (326.5966, 107) -> (326.5966, 106) projected
  line L241 (326.5966, 106) -> (378, 106) projected
  arc A346 (380, 104) -> (378, 106) centre (378, 104) ccw projected
  line L242 (380, 104) -> (380, -104) projected
  arc A347 (378, -106) -> (380, -104) centre (378, -104) ccw projected
  line L243 (378, -106) -> (326.5966, -106) projected
  line L244 (326.5966, -106) -> (326.5966, -107) projected
  line L245 (326.5966, -107) -> (377, -107) projected
  arc A348 (380, -110) -> (377, -107) centre (377, -110) ccw projected
  line L246 (380, -110) -> (417.7779, -195.9889) projected
  arc A349 (413.2002, -203) -> (417.7779, -195.9889) centre (413.2002, -198) ccw projected
  line L247 (413.2002, -203) -> (3, -203) projected
  arc A350 (0, -200) -> (3, -203) centre (3, -200) ccw projected
  line L248 (0, -200) -> (0, 200) projected
  arc A351 (3, 203) -> (0, 200) centre (3, 200) ccw projected
  line L249 (3, 203) -> (413.2002, 203) projected
  point P0 (0, 203)
  point P1 (0, 364.725)
  point P2 (380, 325)
  dimension "d0" = 380
  dimension "d1" = 406
  dimension "d3" = 0
  dimension "d4" = 0
  dimension "d5" = 0
  dimension "d6" = 0
  dimension "d8" = 100
  dimension "d9" = 122
  dimension "d83" = 9.5
  dimension "d84" = 9.5
  dimension "d85" = 0
  dimension "d86" = 0
  dimension "d87" = 0
  dimension "d88" = 0
  dimension "d89" = 0
  constraints: 20 centre point, 18 end point, 11 vertical alignment, 10 equal radius, 3 parallel, 2 midpoint, 2 symmetric about line, 1 horizontal, 1 perpendicular, 1 vertical, 12 other
  measures "d0" distance of L3.start L1.end
  measures "d1" distance of L1.end L1.start
  measures "d3" vertical distance of A4.centre A2.centre
  measures "d4" vertical distance of A2.centre A0.centre
  measures "d5" vertical distance of A0.centre A1.centre
  measures "d6" vertical distance of A1.centre A3.centre
  measures "d8" distance of L8.end L7.end
  measures "d9" distance of L7.end L6.end
  measures "d85" vertical distance of A12.centre A55.centre
  measures "d86" vertical distance of A12.centre A11.centre
  measures "d87" vertical distance of A35.centre A14.centre
  measures "d88" vertical distance of A14.centre A13.centre
  measures "d89" vertical distance of A10.centre A13.centre
extrude "Выдавливание1" add sketch "Эскиз1" along normal blind 1.5 contours L0 A69 L164 A240 A241 A242 L162 A238 L163 A185 L110 L212 A312 L213 L235 A341 L236 A342 L237 A343 L229 A333 L230 A334 L228 A330 L3 A351 L5 L7 L41 A107 L42 A108 L43 L85 A155 L82 A152 L83 A153 L84 L8 L1 L155 A231 L153 A229 A174 L99 A1 A175 L97 L91 A163 A164 A165 L92 A166 | L0 A69 | A166 L92 A165 A164 A163 L91 L0 | L0 L163 A238 L162 A242 A241 A240 L164 | L97 A175 L99 A1 A174 L0 | L0 L110 A185 | A229 L153 A231 L155 L0 | L0 L213 A312 L212 | L0 A343 L237 A342 L236 A341 L235 | L84 A153 L83 A152 L82 A155 L85 L7 L8 | L0 A330 L228 A334 L230 A333 L229 | L11 L10 L5 L3 L2 L1 | L43 A108 L42 A107 L41 L7 | A351 L3 L5 | A0 A234 L158 A233 L157 A232 L156 | A20 | L15 A24 L14 A23 L13 A22 L12 A21 | A30 A29 | A42 A41 | A44 A43 | A46 A45 | A58 A57 | A60 A59 | A65 | A67 | A72 | A76 | A77 | A78 | A84 | A85 | A110 L52 A117 L51 A116 L50 A115 L49 A114 L48 A113 L47 A112 L46 A111 L45 | A120 L55 A119 L54 A118 L53 | A136 L69 A135 L68 A134 L67 | A143 L75 L74 A142 L73 | A148 A147 A146 L78 A145 L77 A144 L76 | L81 A151 L80 A150 L79 A149 | A159 L89 A158 L88 A157 L87 A156 L86 | A184 L108 A183 L107 A182 L106 | A195 L119 A194 L118 A193 L117 A192 L116 | A198 L122 A197 L121 A196 L120 | A207 L131 A206 L130 A205 L129 | A210 L134 A209 L133 A208 L132 | A213 L137 A212 L136 A211 L135 | A217 L141 A216 L140 A215 L139 A214 L138 | A220 L144 A219 L143 A218 L142 | A225 L149 A224 L148 A223 L147 A222 L146 A221 L145 | A255 L175 A254 A253 A252 L174 A251 L173 | A268 L184 A267 L183 A266 L182 | A292 L201 A291 L200 A290 L199 | A298 A297 A296 L204 A295 L203 A294 L202 | A306 L210 A305 L209 A304 L208 | A317 L217 A316 L216 A315 L215 | A320 L220 A319 L219 A318 L218 | A321 A326 L224 A325 L223 A324 L222 A323 L221 A322 | A329 L227 A328 L226 A327 L225 | A340 L234 A339 L233 A338 L232 A337 A336 A335 L231 picked at (134.0397, 0.0074)